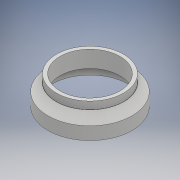
# Autodesk Inventor part: 850_10_filter_holder_v2
Saved by Autodesk Inventor 2018 (Build 220112000, 112)
## iProperties
Created: 2021-07-13
Part Number: 850_10_filter_holder_v2
Material: Generic
Document SubType Name: Modeling
Designer: Gergely Turi
Density: 1 g/cm^3
Appearance: Default
Author: Gergely Turi
Autodesk Inventor part; units mm, degrees
ref_plane "YZ Plane" through (0, 0, 0) normal (1, 0, 0) x (0, 1, 0)
ref_plane "XZ Plane" through (0, 0, 0) normal (0, 1, 0) x (-1, 0, 0)
ref_plane "XY Plane" through (0, 0, 0) normal (0, 0, 1) x (1, 0, 0)
sketch "Sketch1" plane through (0, 0, 0) normal (0, 0, 1) x (1, 0, 0)
  circle A0 centre (0, 0) radius 16.5
  circle A1 centre (0, 0) radius 18.0545
  dimension "d0" = 33
  dimension "d1" = 1.5545
  constraints: 2 centre point, 1 coincident
  measures "d0" diameter of A0
  measures "d1" radial gap between concentric circles of A0 A1
extrude "Extrusion1" add sketch "Sketch1" along normal blind 5
sketch "Sketch4" plane through (0, 0, 5) normal (0, 0, 1) x (1, 0, 0)
  circle A0 centre (0, 0) radius 12.9
  circle A1 centre (0, 0) radius 14.4627
  dimension "d4" = 25.8
  dimension "d5" = 1.5627
  constraints: 2 centre point, 1 coincident
  measures "d4" diameter of A0
  measures "d5" radial gap between concentric circles of A0 A1
extrude "Extrusion2" add sketch "Sketch4" along normal blind 7.2
sketch "Sketch5" plane through (0, 0, 5) normal (0, 0, 1) x (1, 0, 0)
  circle A0 centre (0, 0) radius 18.0545
  circle A1 centre (0, 0) radius 14.2127
  circle A2 centre (0, 0) radius 18.0545 projected
  constraints: 2 centre point, 2 coincident, 1 concentric
extrude "Extrusion3" add sketch "Sketch5" along normal blind 4
chamfer "Chamfer2" distance 3.5 angle 45 1 edges at (-18.0545, 0, 9) measured on face at (16.5423, -2.594, 9)
body "Solid1"
